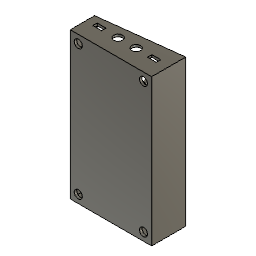
01-petg-body (Autodesk Fusion 360 design; units mm, degrees)
Autodesk Fusion 360 part; units mm, degrees
sketch "Side_Profile_YZ" plane through (0, 0, 0) normal (1, 0, 0) x (0, 0, -1)
  line L0 (0, 0, 0) -> (0, 0, 100)
  line L1 (0, 0, 100) -> (0, 42, 100)
  line L2 (0, 42, 100) -> (0, 30, 0)
  line L3 (0, 30) -> (0, 0)
extrude "Extrude1" add sketch "Side_Profile_YZ" along normal mid plane 180 contours L0 L1 L2 L3 in plane through (0, 0, 0) normal (0, 0, -1)
shell "Shell1" thickness 3 removed faces 1 at (66.6667, 38, 30)
ref_plane "WorkPlane1" through (0, 0, 90) normal (0, 0, 1) x (1, 0, 0)
ref_plane "WorkPlane2" through (0, 0, -90) normal (0, 0, 1) x (1, 0, 0)
ref_plane "WorkPlane3" through (0, 0, 0) normal (1, 0, 0) x (0, 1, 0)
sketch "Cut_R_USBC_Pwr" plane through (0, 0, 90) normal (0, 0, 1) x (1, 0, 0)
  line L0 (9.6, 18.35) -> (20.4, 18.35)
  line L1 (20.4, 18.35) -> (20.4, 23.65)
  line L2 (20.4, 23.65) -> (9.6, 23.65)
  line L3 (9.6, 23.65) -> (9.6, 18.35)
sketch "Cut_R_TRS_OUTL" plane through (0, 0, 90) normal (0, 0, 1) x (1, 0, 0)
  circle A0 centre (38, 21) radius 5.4
sketch "Cut_R_TRS_OUTR" plane through (0, 0, 90) normal (0, 0, 1) x (1, 0, 0)
  circle A0 centre (60, 21) radius 5.4
sketch "Cut_R_USBC_Teen" plane through (0, 0, 90) normal (0, 0, 1) x (1, 0, 0)
  line L0 (74.6, 18.35) -> (85.4, 18.35)
  line L1 (85.4, 18.35) -> (85.4, 23.65)
  line L2 (85.4, 23.65) -> (74.6, 23.65)
  line L3 (74.6, 23.65) -> (74.6, 18.35)
sketch "Cut_R_USBA" plane through (0, 0, 90) normal (0, 0, 1) x (1, 0, 0)
  line L0 (84.35, 16.85) -> (99.65, 16.85)
  line L1 (99.65, 16.85) -> (99.65, 25.15)
  line L2 (99.65, 25.15) -> (84.35, 25.15)
  line L3 (84.35, 25.15) -> (84.35, 16.85)
sketch "Cut_L_TRS_INL" plane through (0, 0, -90) normal (0, 0, 1) x (1, 0, 0)
  circle A0 centre (30, 21) radius 5.4
extrude "Extrude7" cut sketch "Cut_L_TRS_INL" along normal blind 10
sketch "Cut_L_TRS_INR" plane through (0, 0, -90) normal (0, 0, 1) x (1, 0, 0)
  circle A0 centre (55, 21) radius 5.4
extrude "Extrude8" cut sketch "Cut_L_TRS_INR" along normal blind 10
sketch "Cut_L_AUX" plane through (0, 0, -90) normal (0, 0, 1) x (1, 0, 0)
  circle A0 centre (78, 21) radius 3.65
extrude "Extrude9" cut sketch "Cut_L_AUX" along normal blind 10
sketch "Cut_Pogo" plane through (0, 0, 0) normal (1, 0, 0) x (0, 0, -1)
  line L0 (-7.15, 10.85) -> (7.15, 10.85)
  line L1 (7.15, 10.85) -> (7.15, 19.15)
  line L2 (7.15, 19.15) -> (-7.15, 19.15)
  line L3 (-7.15, 19.15) -> (-7.15, 10.85)
extrude "Extrude10" cut sketch "Cut_Pogo" along normal blind 10
ref_plane "WorkPlane4" through (0, 3, 0) normal (0, 1, 0) x (0, 0, 1)
sketch "PCB_Standoffs_OD" plane through (0, 3, 0) normal (0, 1, 0) x (1, 0, 0)
  circle A0 centre (13, -74) radius 3
  circle A1 centre (13, 0) radius 3
  circle A2 centre (13, 74) radius 3
  circle A3 centre (87, -74) radius 3
  circle A4 centre (87, 0) radius 3
  circle A5 centre (87, 74) radius 3
extrude "Extrude11" add sketch "PCB_Standoffs_OD" along normal blind 5
sketch "PCB_Standoffs_M3" plane through (0, 3, 0) normal (0, 1, 0) x (1, 0, 0)
  circle A0 centre (13, -74) radius 2.1
  circle A1 centre (13, 0) radius 2.1
  circle A2 centre (13, 74) radius 2.1
  circle A3 centre (87, -74) radius 2.1
  circle A4 centre (87, 0) radius 2.1
  circle A5 centre (87, 74) radius 2.1
extrude "Extrude12" cut sketch "PCB_Standoffs_M3" along normal blind 6
sketch "Rubber_Feet" plane through (0, 0, 0) normal (0, 1, 0) x (1, 0, 0)
  circle A0 centre (10, -80) radius 4.95
  circle A1 centre (10, 80) radius 4.95
  circle A2 centre (90, -80) radius 4.95
  circle A3 centre (90, 80) radius 4.95
extrude "Extrude13" cut sketch "Rubber_Feet" along normal blind 3
sketch "Cut_R_USBC_Data" plane through (0, 0, 90) normal (0, 0, 1) x (1, 0, 0)
  line L0 (9.6, 18.35) -> (20.4, 18.35)
  line L1 (20.4, 18.35) -> (20.4, 23.65)
  line L2 (20.4, 23.65) -> (9.6, 23.65)
  line L3 (9.6, 23.65) -> (9.6, 18.35)
extrude "Extrude14" cut sketch "Cut_R_USBC_Data" against normal blind 10
sketch "Cut_R_TRS_OUTL (1)" plane through (0, 0, 90) normal (0, 0, 1) x (1, 0, 0)
  circle A0 centre (38, 21) radius 5.4
extrude "Extrude15" cut sketch "Cut_R_TRS_OUTL (1)" against normal blind 10
sketch "Cut_R_TRS_OUTR (1)" plane through (0, 0, 90) normal (0, 0, 1) x (1, 0, 0)
  circle A0 centre (60, 21) radius 5.4
extrude "Extrude16" cut sketch "Cut_R_TRS_OUTR (1)" against normal blind 10
sketch "Cut_R_USBC_Host" plane through (0, 0, 90) normal (0, 0, 1) x (1, 0, 0)
  line L0 (76.6, 18.35) -> (87.4, 18.35)
  line L1 (87.4, 18.35) -> (87.4, 23.65)
  line L2 (87.4, 23.65) -> (76.6, 23.65)
  line L3 (76.6, 23.65) -> (76.6, 18.35)
extrude "Extrude17" cut sketch "Cut_R_USBC_Host" against normal blind 10
named bodies: "PETG_Solid"
